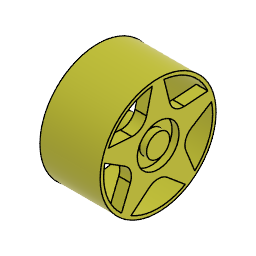
Rim (Autodesk Fusion 360 design; units mm, degrees)
part number: 2026-01-02-23-41-02-488
Autodesk Fusion 360 part; units mm, degrees
sketch "Boceto1" plane through (0, 0, 0) normal (1, 0, 0) x (0, 1, 0)
  circle A0 centre (0, 0) radius 25
  dimension "d1" = 50
  constraint coincident A0.centre origin
  measures "d1" diameter of A0
extrude "Wheel width" add sketch "Boceto1" along normal blind 26
sketch "Boceto2" plane through (26, 0, 0) normal (1, 0, 0) x (0, 1, 0)
  circle A0 centre (0, 0) radius 25
  circle A1 centre (0, 0) radius 5
  circle A2 centre (0, 0) radius 9
  dimension "d4" = 10
  dimension "d5" = 18
  constraint coincident A0.centre A1.centre
  measures "d4" diameter of A1
  measures "d5" diameter of A2
extrude "Wheel profile 1 (1)" cut sketch "Boceto2" against normal blind 3 contours A2
sketch "Boceto3" plane through (26, 0, 0) normal (1, 0, 0) x (0, 1, 0)
  circle A0 centre (0, 0) radius 25
  circle A1 centre (0, 0) radius 9
  circle A2 centre (0, 0) radius 23.5
  line L0 (0, 23.5) -> (0, 13.5) construction
  line L1 (0, 13.5) -> (-5, 13.5)
  line L2 (0, 13.5) -> (5, 13.5)
  line L3 (0, 23.5) -> (-2.5, 23.5)
  line L4 (-2.5, 23.5) -> (-5, 13.5)
  line L5 (2.5, 23.5) -> (5, 13.5)
  line L6 (0, 23.5) -> (2.5, 23.5)
  line L7 (-12.8393, 4.1717) -> (-11.2942, 8.927)
  line L8 (-12.8393, 4.1717) -> (-14.3843, -0.5836)
  line L9 (-23.1224, 4.8843) -> (-14.3843, -0.5836)
  line L10 (-22.3498, 7.2619) -> (-23.1224, 4.8843)
  line L11 (-22.3498, 7.2619) -> (-21.5773, 9.6395)
  line L12 (-21.5773, 9.6395) -> (-11.2942, 8.927)
  line L13 (-7.9351, -10.9217) -> (-11.9802, -7.9828)
  line L14 (-7.9351, -10.9217) -> (-3.89, -13.8607)
  line L15 (-11.7904, -20.4814) -> (-3.89, -13.8607)
  line L16 (-13.813, -19.0119) -> (-11.7904, -20.4814)
  line L17 (-13.813, -19.0119) -> (-15.8355, -17.5424)
  line L18 (-15.8355, -17.5424) -> (-11.9802, -7.9828)
  line L19 (7.9351, -10.9217) -> (3.89, -13.8607)
  line L20 (7.9351, -10.9217) -> (11.9802, -7.9828)
  line L21 (15.8355, -17.5424) -> (11.9802, -7.9828)
  line L22 (13.813, -19.0119) -> (15.8355, -17.5424)
  line L23 (13.813, -19.0119) -> (11.7904, -20.4814)
  line L24 (11.7904, -20.4814) -> (3.89, -13.8607)
  line L25 (12.8393, 4.1717) -> (14.3843, -0.5836)
  line L26 (12.8393, 4.1717) -> (11.2942, 8.927)
  line L27 (21.5773, 9.6395) -> (11.2942, 8.927)
  line L28 (22.3498, 7.2619) -> (21.5773, 9.6395)
  line L29 (22.3498, 7.2619) -> (23.1224, 4.8843)
  line L30 (23.1224, 4.8843) -> (14.3843, -0.5836)
  arc A3 (-11.2942, 8.927) -> (-5, 13.5) centre (-10.8755, 14.9689) ccw
  arc A4 (-11.9802, -7.9828) -> (-14.3843, -0.5836) centre (-17.597, -5.7176) ccw
  arc A5 (3.89, -13.8607) -> (-3.89, -13.8607) centre (0, -18.5026) ccw
  arc A6 (14.3843, -0.5836) -> (11.9802, -7.9828) centre (17.597, -5.7176) ccw
  arc A7 (5, 13.5) -> (11.2942, 8.927) centre (10.8755, 14.9689) ccw
  dimension "d8" = 47
  dimension "d9" = 10
  dimension "d10" = 5
  dimension "d12" = 2.5
  dimension "d14" = 360
  constraint coincident A0.centre A1.centre
  constraint coincident A2 L0.start
  constraint vertical L0
  constraint perpendicular L0 L1
  constraint symmetric L1.start L0 L2.start
  constraint symmetric L0 L1.end L2.end
  constraint perpendicular L0 L3
  constraint symmetric L3.start L0 L6.start
  constraint symmetric L0 L3.end L5.start
  constraint tangent L4 A3
  constraint tangent L9 A4
  constraint tangent L15 A5
  constraint tangent L21 A6
  constraint tangent L27 A7
  measures "d8" diameter of A2
  measures "d9" distance of L0.start L0.end
  measures "d10" distance of L0.end L1.end
  measures "d12" distance of L0.start L3.end
extrude "Wheel profile 2 (1)" cut sketch "Boceto3" against normal through all contours A2 L21 L30 A6 | A2 L5 L27 A7 | A2 L15 L24 A5 | A2 L4 L12 A3 | A2 L9 L18 A4
sketch "Boceto4" plane through (0, 0, 0) normal (-1, 0, 0) x (0, -1, 0)
  line L0 (-11.9802, -7.9828) -> (-15.7827, -17.4114)
  arc A0 (-23.0026, 4.8093) -> (-15.7827, -17.4114) centre (0, 0) ccw
  line L1 (-23.0026, 4.8093) -> (-14.3843, -0.5836)
  arc A1 (-11.9802, -7.9828) -> (-14.3843, -0.5836) centre (-17.597, -5.7176) ccw
  line L2 (-11.2942, 8.927) -> (-21.4364, 9.6298)
  arc A2 (-2.5343, 23.363) -> (-21.4364, 9.6298) centre (0, 0) ccw
  line L3 (-2.5343, 23.363) -> (-5, 13.5)
  arc A3 (-11.2942, 8.927) -> (-5, 13.5) centre (-10.8755, 14.9689) ccw
  line L4 (3.89, -13.8607) -> (11.6821, -20.3906)
  arc A4 (-11.6821, -20.3906) -> (11.6821, -20.3906) centre (0, 0) ccw
  line L5 (-11.6821, -20.3906) -> (-3.89, -13.8607)
  arc A5 (3.89, -13.8607) -> (-3.89, -13.8607) centre (0, -18.5026) ccw
  line L6 (5, 13.5) -> (2.5343, 23.363)
  arc A6 (21.4364, 9.6298) -> (2.5343, 23.363) centre (0, 0) ccw
  line L7 (21.4364, 9.6298) -> (11.2942, 8.927)
  arc A7 (5, 13.5) -> (11.2942, 8.927) centre (10.8755, 14.9689) ccw
  line L8 (14.3843, -0.5836) -> (23.0026, 4.8093)
  arc A8 (15.7827, -17.4114) -> (23.0026, 4.8093) centre (0, 0) ccw
  line L9 (15.7827, -17.4114) -> (11.9802, -7.9828)
  arc A9 (14.3843, -0.5836) -> (11.9802, -7.9828) centre (17.597, -5.7176) ccw
  circle A10 centre (0, 0) radius 25
  circle A11 centre (0, 0) radius 23.5
  constraint coincident A0.centre A2.centre
extrude "Wheel hole (1)" cut sketch "Boceto4" against normal blind 21 contours L0 L1 A1 L2 L3 A3 L4 L5 A5 L6 L7 A7 L8 L9 A9 A11
sketch "Boceto5" plane through (21, 0, 0) normal (-1, 0, 0) x (0, -1, 0)
  line L0 (3.89, -13.8607) -> (11.6821, -20.3906)
  arc A0 (11.6821, -20.3906) -> (15.7827, -17.4114) centre (0, 0) ccw
  line L1 (15.7827, -17.4114) -> (11.9802, -7.9828)
  arc A1 (14.3843, -0.5836) -> (11.9802, -7.9828) centre (17.597, -5.7176) ccw
  line L2 (14.3843, -0.5836) -> (23.0026, 4.8093)
  arc A2 (23.0026, 4.8093) -> (21.4364, 9.6298) centre (0, 0) ccw
  line L3 (21.4364, 9.6298) -> (11.2942, 8.927)
  arc A3 (5, 13.5) -> (11.2942, 8.927) centre (10.8755, 14.9689) ccw
  line L4 (5, 13.5) -> (2.5343, 23.363)
  arc A4 (2.5343, 23.363) -> (-2.5343, 23.363) centre (0, 0) ccw
  line L5 (-2.5343, 23.363) -> (-5, 13.5)
  arc A5 (-11.2942, 8.927) -> (-5, 13.5) centre (-10.8755, 14.9689) ccw
  line L6 (-11.2942, 8.927) -> (-21.4364, 9.6298)
  arc A6 (-21.4364, 9.6298) -> (-23.0026, 4.8093) centre (0, 0) ccw
  line L7 (-23.0026, 4.8093) -> (-14.3843, -0.5836)
  arc A7 (-11.9802, -7.9828) -> (-14.3843, -0.5836) centre (-17.597, -5.7176) ccw
  line L8 (-11.9802, -7.9828) -> (-15.7827, -17.4114)
  arc A8 (-15.7827, -17.4114) -> (-11.6821, -20.3906) centre (0, 0) ccw
  line L9 (-11.6821, -20.3906) -> (-3.89, -13.8607)
  arc A9 (3.89, -13.8607) -> (-3.89, -13.8607) centre (0, -18.5026) ccw
  circle A10 centre (0, 0) radius 5
  dimension "d18" = 10
  constraint coincident A0.centre A2.centre
  measures "d18" diameter of A10
extrude "Connector base (1)" add sketch "Boceto5" along normal blind 10 contours A10
sketch "Boceto6" plane through (11, 0, 0) normal (-1, 0, 0) x (0, -1, 0)
  circle A0 centre (0, 0) radius 5
  line L0 (1.85, 1.9666) -> (-1.85, 1.9666)
  line L1 (-1.85, -1.9666) -> (1.85, -1.9666)
  arc A1 (-1.85, 1.9666) -> (-1.85, -1.9666) centre (0, 0) ccw
  arc A2 (1.85, -1.9666) -> (1.85, 1.9666) centre (0, 0) ccw
  dimension "d21" = 5.4
  dimension "d22" = 3.7
  constraint coincident A0.centre A1.centre
  constraint horizontal L0
  constraint parallel L0 L1
  constraint concentric A1 A2
  measures "d21" diameter of A1
  measures "d22" distance of L0.start L0.end
extrude "Connector hole (1)" cut sketch "Boceto6" against normal blind 9 contours L0 L1 A1 A2
named bodies: "Wheel"
